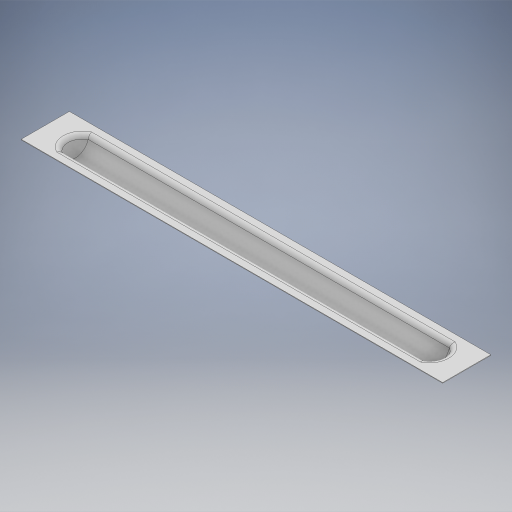
# Autodesk Inventor part: A2.2-long-punch-3
Saved by Autodesk Inventor 2024 (Build 280153000, 153)
## iProperties
Created: 2024-02-18
Part Number: A2.2-long-punch-3
Material: Generic
Document SubType Name: Sheet Metal
Designer: Alex
Density: 1 g/cm^3
Sheet Metal Rule: Default_mm
Appearance: Default
Author: Alex
Autodesk Inventor part; units mm, degrees
ref_plane "YZ Plane" through (0, 0, 0) normal (1, 0, 0) x (0, 1, 0)
ref_plane "XZ Plane" through (0, 0, 0) normal (0, 1, 0) x (-1, 0, 0)
ref_plane "XY Plane" through (0, 0, 0) normal (0, 0, 1) x (1, 0, 0)
sketch "Sketch1" plane through (0, 0, 0) normal (0, 1, 0) x (-1, 0, 0)
  line L0 (0, 0) -> (-350, 0)
  line L1 (-350, 0) -> (-350, -40)
  line L2 (-350, -40) -> (0, -40)
  line L3 (0, -40) -> (0, 0)
  dimension "d0" = 350
  dimension "d1" = 40
  measures "d0" distance of L2.end L1.end
  measures "d1" distance of L1.end L0.end
extrude "Plate1" add sketch "Sketch1" along normal blind 0.5
sketch "Sketch2" plane through (0, 0.5, 0) normal (0, 1, 0) x (1, 0, 0)
  line L0 (25, 31) -> (325, 31)
  line L1 (25, 9) -> (325, 9)
  line L2 (18.4372, 20) -> (331.5628, 20) construction
  arc A0 (325, 9) -> (325, 31) centre (319.0628, 20) ccw
  line L3 (319.0628, 6.0647) -> (319.0628, 33.9353) construction
  line L4 (175, 9) -> (175, 31) construction
  arc A1 (25, 31) -> (25, 9) centre (30.9372, 20) ccw
  line L5 (30.9372, 6.0647) -> (30.9372, 33.9353) construction
  line L6 (350, 0) -> (0, 0) construction
  line L7 (0, 0) -> (0, 40) construction
  arc A2 (24.5146, 33) -> (16.4372, 20) centre (30.9372, 20) ccw
  line L8 (24.5146, 33) -> (325.4854, 33)
  arc A3 (333.5628, 20) -> (325.4854, 33) centre (319.0628, 20) ccw
  line L9 (331.5628, 20) -> (333.5628, 20)
  line L10 (18.4372, 20) -> (16.4372, 20)
  point P0 (25, 20)
  point P1 (325, 20)
  point P2 (319.0628, 20)
  point P3 (175, 20)
  dimension "d4" = 22
  dimension "d5" = 300
  dimension "d6" = 25
  dimension "d7" = 22
  dimension "d8" = 20
  dimension "d9" = 175
  dimension "d16" = 2
  dimension "d17" = 2
  dimension "d18" = 2
  constraints: 18 end point, 12 point on circle, 6 midpoint, 5 horizontal, 4 centre point, 4 vertical alignment, 3 point on line, 3 symmetric about line, 2 concentric, 1 perpendicular, 1 vertical, 1 other
  measures "d4" distance between parallel lines of L1 L0
  measures "d5" distance of L0.end L0.start
  measures "d6" diameter of A0
  measures "d7" diameter of L0 L2
  measures "d8" distance from line of L6 point (175, 20)
  measures "d9" distance from line of L7 point (175, 20)
  measures "d16" distance of L10.start L10.end
  measures "d17" distance of L9.start L9.end
  measures "d18" distance between parallel lines of L0 L8
extrude "Extrusion1" cut sketch "Sketch2" against normal blind 0.5 contours L0 A0 L1 A1
revolve "Revolution1" add sketch "Sketch2" angle 180 about axis through (18.4372, 0.5, -20) along (-1, 0, 0) contours A1 L10 A2 L8 A3 L9 A0 L0
fillet "Fillet1" radius 4 10 edges at (175, 0.5, -31) (175, 0.5, -9) (20.2025, 0.5, -26.4045) (20.2025, 0.5, -13.5955) (329.7975, 0.5, -26.4045) (329.7975, 0.5, -13.5955) (175, 0, -7.0096) (175, 0, -32.9904) (333.5542, 0, -20) (16.4458, 0, -20)
equation "\"d16\" = 4 * Thickness"
equation "\"d17\" = 4 * Thickness"
equation "\"d18\" = 4 * Thickness"
equation "\"d10\" = Thickness"
equation "\"d2\" = Thickness"
equation "\"BendRadius\" = Thickness"
equation "\"BendReliefWidth\" = Thickness"
equation "\"BendReliefDepth\" = 0.5 * Thickness"
equation "\"CornerReliefSize\" = 4 * Thickness"
equation "\"MinimumRemnant\" = 2 * Thickness"
equation "\"TransitionRadius\" = BendRadius"
equation "\"JacobiRadiusSize\" = BendRadius"
equation "\"GapSize\" = Thickness"
equation "\"Thickness\" = 0.5"
body "Solid1"
